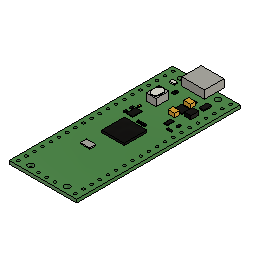
Raspberry+Pi+Pico (Autodesk Fusion 360 design; units mm, degrees)
Autodesk Fusion 360 part; units mm, degrees
sketch "Sketch1" plane through (0, 0, 0) normal (0, 0, 1) x (1, 0, 0)
  point P0 (-8.0088, 19.3196)
  point P1 (-8.0088, -20.4887)
  constraint vertical P0 P1
sketch "Sketch2" plane through (0, 0, 0) normal (0, 0, 1) x (1, 0, 0)
  line L0 (-10.4385, 24.6601) -> (10.5024, 24.6601)
  line L1 (10.5024, 24.6601) -> (10.5024, -25.9245)
  line L2 (10.5024, -25.9245) -> (-10.4385, -25.9245)
  line L3 (-10.4385, -25.9245) -> (-10.4385, 24.6601)
  dimension "d1" = 20.941
  constraint horizontal L0
  constraint vertical L1
  constraint horizontal L2
  constraint vertical L3
  measures "d1" distance of L0.start L0.end
extrude "Extrude1" add sketch "Sketch2" along normal blind 1
extrude "Extrude2" add 1 faces at (3.5221, -25.9245, 0.6667) along direction (0, -1, 0) blind 0.1
extrude "Extrude3" add 1 faces at (3.5221, -26.0245, 0.6667) along direction (0, -1, 0) blind 0.1
sketch "Sketch3" plane through (0, 0, 1) normal (0, 0, 1) x (-1, 0, 0)
  line L0 (-10.5024, 26.1245) -> (-10.5024, -24.6601)
  line L1 (-10.5024, -24.6601) -> (10.4385, -24.6601)
  line L2 (10.4385, -24.6601) -> (10.4385, 26.1245)
  line L3 (10.4385, 26.1245) -> (-10.5024, 26.1245)
  line L4 (3.5791, -2.7776) -> (-3.425, -2.7776)
  line L5 (-3.425, -2.7776) -> (-3.425, 4.2707)
  line L6 (-3.425, 4.2707) -> (3.5791, 4.2707)
  line L7 (3.5791, 4.2707) -> (3.5791, -2.7776)
  constraint horizontal L4
  constraint vertical L5
  constraint horizontal L6
  constraint vertical L7
extrude "Extrude4" add sketch "Sketch3" along normal blind 0.5 contours L4 L5 L6 L7
sketch "Sketch4" plane through (0, 0, 1) normal (0, 0, 1) x (-1, 0, 0)
  line L0 (3.5791, 4.2707) -> (3.5791, -2.7776)
  line L1 (3.5791, -2.7776) -> (-3.425, -2.7776)
  line L2 (-3.425, -2.7776) -> (-3.425, 4.2707)
  line L3 (-3.425, 4.2707) -> (3.5791, 4.2707)
  line L4 (-10.5024, 26.1245) -> (-10.5024, -24.6601)
  line L5 (-10.5024, -24.6601) -> (10.4385, -24.6601)
  line L6 (10.4385, -24.6601) -> (10.4385, 26.1245)
  line L7 (10.4385, 26.1245) -> (-10.5024, 26.1245)
  circle A0 centre (-8.7965, 24.8249) radius 0.4145
  circle A1 centre (-8.7965, 22.288) radius 0.4145
  circle A2 centre (-8.7965, 19.7512) radius 0.4145
  circle A3 centre (-8.7965, 17.2144) radius 0.4145
  circle A4 centre (-8.7965, 14.6775) radius 0.4145
  circle A5 centre (-8.7965, 12.1407) radius 0.4145
  circle A6 centre (-8.7965, 9.6038) radius 0.4145
  circle A7 centre (-8.7965, 7.067) radius 0.4145
  circle A8 centre (-8.7965, 4.5301) radius 0.4145
  circle A9 centre (-8.7965, 1.9933) radius 0.4145
  circle A10 centre (-8.7965, -0.5435) radius 0.4145
  circle A11 centre (-8.7965, -3.0804) radius 0.4145
  circle A12 centre (-8.7965, -5.6172) radius 0.4145
  circle A13 centre (-8.7965, -8.1541) radius 0.4145
  circle A14 centre (-8.7965, -10.6909) radius 0.4145
  circle A15 centre (-8.7965, -13.2277) radius 0.4145
  circle A16 centre (-8.7965, -15.7646) radius 0.4145
  circle A17 centre (-8.7965, -18.3014) radius 0.4145
  circle A18 centre (-8.7965, -20.8383) radius 0.4145
  circle A19 centre (-8.7965, -23.3751) radius 0.4145
  dimension "d10" = 0.829
  dimension "d13" = 0
  dimension "d14" = -48.2
  measures "d10" diameter of A0
extrude "Extrude5" cut sketch "Sketch4" against normal blind 14 contours A0 | A1 | A2 | A3 | A4 | A5 | A6 | A7 | A8 | A9 | A10 | A11 | A12 | A13 | A14 | A15 | A16 | A17 | A18 | A19
sketch "Sketch5" plane through (0, 0, 1) normal (0, 0, 1) x (-1, 0, 0)
  circle A0 centre (-8.7965, -18.3014) radius 0.4145
  circle A1 centre (-8.7965, -8.1541) radius 0.4145
  circle A2 centre (-8.7965, 1.9933) radius 0.4145
  circle A3 centre (-8.7965, 14.6775) radius 0.4145
  circle A4 centre (-8.7965, 24.8249) radius 0.4145
  circle A5 centre (-8.7965, 22.288) radius 0.4145
  circle A6 centre (-8.7965, 12.1407) radius 0.4145
  circle A7 centre (-8.7965, -0.5435) radius 0.4145
  circle A8 centre (-8.7965, -10.6909) radius 0.4145
  circle A9 centre (-8.7965, -20.8383) radius 0.4145
  circle A10 centre (-8.7965, -15.7646) radius 0.4145
  circle A11 centre (-8.7965, -5.6172) radius 0.4145
  circle A12 centre (-8.7965, 7.067) radius 0.4145
  circle A13 centre (-8.7965, 17.2144) radius 0.4145
  circle A14 centre (-8.7965, 4.5301) radius 0.4145
  circle A15 centre (-8.7965, 19.7512) radius 0.4145
  circle A16 centre (-8.7965, 9.6038) radius 0.4145
  circle A17 centre (-8.7965, -3.0804) radius 0.4145
  circle A18 centre (-8.7965, -13.2277) radius 0.4145
  circle A19 centre (-8.7965, -23.3751) radius 0.4145
  line L0 (3.5791, 4.2707) -> (3.5791, -2.7776)
  line L1 (3.5791, -2.7776) -> (-3.425, -2.7776)
  line L2 (-3.425, -2.7776) -> (-3.425, 4.2707)
  line L3 (-3.425, 4.2707) -> (3.5791, 4.2707)
  line L4 (-10.5024, 26.1245) -> (-10.5024, -24.6601)
  line L5 (-10.5024, -24.6601) -> (10.4385, -24.6601)
  line L6 (10.4385, -24.6601) -> (10.4385, 26.1245)
  line L7 (10.4385, 26.1245) -> (-10.5024, 26.1245)
  circle A20 centre (8.9761, 24.8199) radius 0.4252
  circle A21 centre (8.9761, 22.283) radius 0.4252
  circle A22 centre (8.9761, 19.7462) radius 0.4252
  circle A23 centre (8.9761, 17.2093) radius 0.4252
  circle A24 centre (8.9761, 14.6725) radius 0.4252
  circle A25 centre (8.9761, 12.1357) radius 0.4252
  circle A26 centre (8.9761, 9.5988) radius 0.4252
  circle A27 centre (8.9761, 7.062) radius 0.4252
  circle A28 centre (8.9761, 4.5251) radius 0.4252
  circle A29 centre (8.9761, 1.9883) radius 0.4252
  circle A30 centre (8.9761, -0.5486) radius 0.4252
  circle A31 centre (8.9761, -3.0854) radius 0.4252
  circle A32 centre (8.9761, -5.6222) radius 0.4252
  circle A33 centre (8.9761, -8.1591) radius 0.4252
  circle A34 centre (8.9761, -10.6959) radius 0.4252
  circle A35 centre (8.9761, -13.2328) radius 0.4252
  circle A36 centre (8.9761, -15.7696) radius 0.4252
  circle A37 centre (8.9761, -18.3065) radius 0.4252
  circle A38 centre (8.9761, -20.8433) radius 0.4252
  circle A39 centre (8.9761, -23.3801) radius 0.4252
  dimension "d17" = 0.8503
  dimension "d20" = 0
  dimension "d21" = -48.2
  measures "d17" diameter of A20
extrude "Extrude6" cut sketch "Sketch5" against normal blind 1 contours A20 | A21 | A22 | A23 | A24 | A25 | A26 | A27 | A28 | A29 | A30 | A31 | A32 | A33 | A34 | A35 | A36 | A37 | A38 | A39
sketch "Sketch6" plane through (0, 0, 1) normal (0, 0, 1) x (-1, 0, 0)
  circle A0 centre (8.9761, -18.3065) radius 0.4252
  circle A1 centre (8.9761, -8.1591) radius 0.4252
  circle A2 centre (8.9761, 1.9883) radius 0.4252
  circle A3 centre (8.9761, 12.1357) radius 0.4252
  circle A4 centre (8.9761, 22.283) radius 0.4252
  circle A5 centre (8.9761, 19.7462) radius 0.4252
  circle A6 centre (8.9761, 9.5988) radius 0.4252
  circle A7 centre (8.9761, -0.5486) radius 0.4252
  circle A8 centre (8.9761, -10.6959) radius 0.4252
  circle A9 centre (8.9761, -20.8433) radius 0.4252
  circle A10 centre (8.9761, -15.7696) radius 0.4252
  circle A11 centre (8.9761, -5.6222) radius 0.4252
  circle A12 centre (8.9761, 4.5251) radius 0.4252
  circle A13 centre (8.9761, 14.6725) radius 0.4252
  circle A14 centre (8.9761, 24.8199) radius 0.4252
  circle A15 centre (8.9761, 17.2093) radius 0.4252
  circle A16 centre (8.9761, 7.062) radius 0.4252
  circle A17 centre (8.9761, -3.0854) radius 0.4252
  circle A18 centre (8.9761, -13.2328) radius 0.4252
  circle A19 centre (8.9761, -23.3801) radius 0.4252
  circle A20 centre (-8.7965, -18.3014) radius 0.4145
  circle A21 centre (-8.7965, -8.1541) radius 0.4145
  circle A22 centre (-8.7965, 1.9933) radius 0.4145
  circle A23 centre (-8.7965, 14.6775) radius 0.4145
  circle A24 centre (-8.7965, 24.8249) radius 0.4145
  circle A25 centre (-8.7965, 22.288) radius 0.4145
  circle A26 centre (-8.7965, 12.1407) radius 0.4145
  circle A27 centre (-8.7965, -0.5435) radius 0.4145
  circle A28 centre (-8.7965, -10.6909) radius 0.4145
  circle A29 centre (-8.7965, -20.8383) radius 0.4145
  circle A30 centre (-8.7965, -15.7646) radius 0.4145
  circle A31 centre (-8.7965, -5.6172) radius 0.4145
  circle A32 centre (-8.7965, 7.067) radius 0.4145
  circle A33 centre (-8.7965, 17.2144) radius 0.4145
  circle A34 centre (-8.7965, 4.5301) radius 0.4145
  circle A35 centre (-8.7965, 19.7512) radius 0.4145
  circle A36 centre (-8.7965, 9.6038) radius 0.4145
  circle A37 centre (-8.7965, -3.0804) radius 0.4145
  circle A38 centre (-8.7965, -13.2277) radius 0.4145
  circle A39 centre (-8.7965, -23.3751) radius 0.4145
  line L0 (3.5791, 4.2707) -> (3.5791, -2.7776)
  line L1 (3.5791, -2.7776) -> (-3.425, -2.7776)
  line L2 (-3.425, -2.7776) -> (-3.425, 4.2707)
  line L3 (-3.425, 4.2707) -> (3.5791, 4.2707)
  line L4 (-10.5024, 26.1245) -> (-10.5024, -24.6601)
  line L5 (-10.5024, -24.6601) -> (10.4385, -24.6601)
  line L6 (10.4385, -24.6601) -> (10.4385, 26.1245)
  line L7 (10.4385, 26.1245) -> (-10.5024, 26.1245)
  circle A40 centre (-5.6173, 24.1526) radius 0.8768
  circle A41 centre (5.7716, 24.1573) radius 0.8814
extrude "Extrude7" cut sketch "Sketch6" against normal blind 1 contours A40 | A41
sketch "Sketch7" plane through (0, 0, 1) normal (0, 0, 1) x (-1, 0, 0)
  circle A0 centre (-5.6173, 24.1526) radius 0.8768
  circle A1 centre (5.7716, 24.1573) radius 0.8814
  circle A2 centre (8.9761, -18.3065) radius 0.4252
  circle A3 centre (8.9761, -8.1591) radius 0.4252
  circle A4 centre (8.9761, 1.9883) radius 0.4252
  circle A5 centre (8.9761, 12.1357) radius 0.4252
  circle A6 centre (8.9761, 22.283) radius 0.4252
  circle A7 centre (8.9761, 19.7462) radius 0.4252
  circle A8 centre (8.9761, 9.5988) radius 0.4252
  circle A9 centre (8.9761, -0.5486) radius 0.4252
  circle A10 centre (8.9761, -10.6959) radius 0.4252
  circle A11 centre (8.9761, -20.8433) radius 0.4252
  circle A12 centre (8.9761, -15.7696) radius 0.4252
  circle A13 centre (8.9761, -5.6222) radius 0.4252
  circle A14 centre (8.9761, 4.5251) radius 0.4252
  circle A15 centre (8.9761, 14.6725) radius 0.4252
  circle A16 centre (8.9761, 24.8199) radius 0.4252
  circle A17 centre (8.9761, 17.2093) radius 0.4252
  circle A18 centre (8.9761, 7.062) radius 0.4252
  circle A19 centre (8.9761, -3.0854) radius 0.4252
  circle A20 centre (8.9761, -13.2328) radius 0.4252
  circle A21 centre (8.9761, -23.3801) radius 0.4252
  circle A22 centre (-8.7965, -18.3014) radius 0.4145
  circle A23 centre (-8.7965, -8.1541) radius 0.4145
  circle A24 centre (-8.7965, 1.9933) radius 0.4145
  circle A25 centre (-8.7965, 14.6775) radius 0.4145
  circle A26 centre (-8.7965, 24.8249) radius 0.4145
  circle A27 centre (-8.7965, 22.288) radius 0.4145
  circle A28 centre (-8.7965, 12.1407) radius 0.4145
  circle A29 centre (-8.7965, -0.5435) radius 0.4145
  circle A30 centre (-8.7965, -10.6909) radius 0.4145
  circle A31 centre (-8.7965, -20.8383) radius 0.4145
  circle A32 centre (-8.7965, -15.7646) radius 0.4145
  circle A33 centre (-8.7965, -5.6172) radius 0.4145
  circle A34 centre (-8.7965, 7.067) radius 0.4145
  circle A35 centre (-8.7965, 17.2144) radius 0.4145
  circle A36 centre (-8.7965, 4.5301) radius 0.4145
  circle A37 centre (-8.7965, 19.7512) radius 0.4145
  circle A38 centre (-8.7965, 9.6038) radius 0.4145
  circle A39 centre (-8.7965, -3.0804) radius 0.4145
  circle A40 centre (-8.7965, -13.2277) radius 0.4145
  circle A41 centre (-8.7965, -23.3751) radius 0.4145
  line L0 (3.5791, 4.2707) -> (3.5791, -2.7776)
  line L1 (3.5791, -2.7776) -> (-3.425, -2.7776)
  line L2 (-3.425, -2.7776) -> (-3.425, 4.2707)
  line L3 (-3.425, 4.2707) -> (3.5791, 4.2707)
  line L4 (-10.5024, 26.1245) -> (-10.5024, -24.6601)
  line L5 (-10.5024, -24.6601) -> (10.4385, -24.6601)
  line L6 (10.4385, -24.6601) -> (10.4385, 26.1245)
  line L7 (10.4385, 26.1245) -> (-10.5024, 26.1245)
  circle A42 centre (-5.6142, -22.6811) radius 0.8718
  circle A43 centre (5.7752, -22.6811) radius 0.8763
extrude "Extrude8" cut sketch "Sketch7" against normal blind 1 contours A42 | A43
sketch "Sketch8" plane through (0, 0, 1) normal (0, 0, 1) x (-1, 0, 0)
  circle A0 centre (5.7752, -22.6811) radius 0.8763
  circle A1 centre (-5.6142, -22.6811) radius 0.8718
  circle A2 centre (-5.6173, 24.1526) radius 0.8768
  circle A3 centre (5.7716, 24.1573) radius 0.8814
  circle A4 centre (8.9761, -18.3065) radius 0.4252
  circle A5 centre (8.9761, -8.1591) radius 0.4252
  circle A6 centre (8.9761, 1.9883) radius 0.4252
  circle A7 centre (8.9761, 12.1357) radius 0.4252
  circle A8 centre (8.9761, 22.283) radius 0.4252
  circle A9 centre (8.9761, 19.7462) radius 0.4252
  circle A10 centre (8.9761, 9.5988) radius 0.4252
  circle A11 centre (8.9761, -0.5486) radius 0.4252
  circle A12 centre (8.9761, -10.6959) radius 0.4252
  circle A13 centre (8.9761, -20.8433) radius 0.4252
  circle A14 centre (8.9761, -15.7696) radius 0.4252
  circle A15 centre (8.9761, -5.6222) radius 0.4252
  circle A16 centre (8.9761, 4.5251) radius 0.4252
  circle A17 centre (8.9761, 14.6725) radius 0.4252
  circle A18 centre (8.9761, 24.8199) radius 0.4252
  circle A19 centre (8.9761, 17.2093) radius 0.4252
  circle A20 centre (8.9761, 7.062) radius 0.4252
  circle A21 centre (8.9761, -3.0854) radius 0.4252
  circle A22 centre (8.9761, -13.2328) radius 0.4252
  circle A23 centre (8.9761, -23.3801) radius 0.4252
  circle A24 centre (-8.7965, -18.3014) radius 0.4145
  circle A25 centre (-8.7965, -8.1541) radius 0.4145
  circle A26 centre (-8.7965, 1.9933) radius 0.4145
  circle A27 centre (-8.7965, 14.6775) radius 0.4145
  circle A28 centre (-8.7965, 24.8249) radius 0.4145
  circle A29 centre (-8.7965, 22.288) radius 0.4145
  circle A30 centre (-8.7965, 12.1407) radius 0.4145
  circle A31 centre (-8.7965, -0.5435) radius 0.4145
  circle A32 centre (-8.7965, -10.6909) radius 0.4145
  circle A33 centre (-8.7965, -20.8383) radius 0.4145
  circle A34 centre (-8.7965, -15.7646) radius 0.4145
  circle A35 centre (-8.7965, -5.6172) radius 0.4145
  circle A36 centre (-8.7965, 7.067) radius 0.4145
  circle A37 centre (-8.7965, 17.2144) radius 0.4145
  circle A38 centre (-8.7965, 4.5301) radius 0.4145
  circle A39 centre (-8.7965, 19.7512) radius 0.4145
  circle A40 centre (-8.7965, 9.6038) radius 0.4145
  circle A41 centre (-8.7965, -3.0804) radius 0.4145
  circle A42 centre (-8.7965, -13.2277) radius 0.4145
  circle A43 centre (-8.7965, -23.3751) radius 0.4145
  line L0 (3.5791, 4.2707) -> (3.5791, -2.7776)
  line L1 (3.5791, -2.7776) -> (-3.425, -2.7776)
  line L2 (-3.425, -2.7776) -> (-3.425, 4.2707)
  line L3 (-3.425, 4.2707) -> (3.5791, 4.2707)
  line L4 (-10.5024, 26.1245) -> (-10.5024, -24.6601)
  line L5 (-10.5024, -24.6601) -> (10.4385, -24.6601)
  line L6 (10.4385, -24.6601) -> (10.4385, 26.1245)
  line L7 (10.4385, 26.1245) -> (-10.5024, 26.1245)
  circle A44 centre (-2.4417, 24.8384) radius 0.4303
  circle A45 centre (0.0875, 24.8217) radius 0.4265
  circle A46 centre (2.6066, 24.8384) radius 0.43
extrude "Extrude9" cut sketch "Sketch8" against normal blind 1 contours A44 | A45 | A46
sketch "Sketch9" plane through (0, 0, 1) normal (0, 0, 1) x (-1, 0, 0)
  circle A0 centre (2.6066, 24.8384) radius 0.43
  circle A1 centre (0.0875, 24.8217) radius 0.4265
  circle A2 centre (-2.4417, 24.8384) radius 0.4303
  circle A3 centre (5.7752, -22.6811) radius 0.8763
  circle A4 centre (-5.6142, -22.6811) radius 0.8718
  circle A5 centre (-5.6173, 24.1526) radius 0.8768
  circle A6 centre (5.7716, 24.1573) radius 0.8814
  circle A7 centre (8.9761, -18.3065) radius 0.4252
  circle A8 centre (8.9761, -8.1591) radius 0.4252
  circle A9 centre (8.9761, 1.9883) radius 0.4252
  circle A10 centre (8.9761, 12.1357) radius 0.4252
  circle A11 centre (8.9761, 22.283) radius 0.4252
  circle A12 centre (8.9761, 19.7462) radius 0.4252
  circle A13 centre (8.9761, 9.5988) radius 0.4252
  circle A14 centre (8.9761, -0.5486) radius 0.4252
  circle A15 centre (8.9761, -10.6959) radius 0.4252
  circle A16 centre (8.9761, -20.8433) radius 0.4252
  circle A17 centre (8.9761, -15.7696) radius 0.4252
  circle A18 centre (8.9761, -5.6222) radius 0.4252
  circle A19 centre (8.9761, 4.5251) radius 0.4252
  circle A20 centre (8.9761, 14.6725) radius 0.4252
  circle A21 centre (8.9761, 24.8199) radius 0.4252
  circle A22 centre (8.9761, 17.2093) radius 0.4252
  circle A23 centre (8.9761, 7.062) radius 0.4252
  circle A24 centre (8.9761, -3.0854) radius 0.4252
  circle A25 centre (8.9761, -13.2328) radius 0.4252
  circle A26 centre (8.9761, -23.3801) radius 0.4252
  circle A27 centre (-8.7965, -18.3014) radius 0.4145
  circle A28 centre (-8.7965, -8.1541) radius 0.4145
  circle A29 centre (-8.7965, 1.9933) radius 0.4145
  circle A30 centre (-8.7965, 14.6775) radius 0.4145
  circle A31 centre (-8.7965, 24.8249) radius 0.4145
  circle A32 centre (-8.7965, 22.288) radius 0.4145
  circle A33 centre (-8.7965, 12.1407) radius 0.4145
  circle A34 centre (-8.7965, -0.5435) radius 0.4145
  circle A35 centre (-8.7965, -10.6909) radius 0.4145
  circle A36 centre (-8.7965, -20.8383) radius 0.4145
  circle A37 centre (-8.7965, -15.7646) radius 0.4145
  circle A38 centre (-8.7965, -5.6172) radius 0.4145
  circle A39 centre (-8.7965, 7.067) radius 0.4145
  circle A40 centre (-8.7965, 17.2144) radius 0.4145
  circle A41 centre (-8.7965, 4.5301) radius 0.4145
  circle A42 centre (-8.7965, 19.7512) radius 0.4145
  circle A43 centre (-8.7965, 9.6038) radius 0.4145
  circle A44 centre (-8.7965, -3.0804) radius 0.4145
  circle A45 centre (-8.7965, -13.2277) radius 0.4145
  circle A46 centre (-8.7965, -23.3751) radius 0.4145
  line L0 (3.5791, 4.2707) -> (3.5791, -2.7776)
  line L1 (3.5791, -2.7776) -> (-3.425, -2.7776)
  line L2 (-3.425, -2.7776) -> (-3.425, 4.2707)
  line L3 (-3.425, 4.2707) -> (3.5791, 4.2707)
  line L4 (-10.5024, 26.1245) -> (-10.5024, -24.6601)
  line L5 (-10.5024, -24.6601) -> (10.4385, -24.6601)
  line L6 (10.4385, -24.6601) -> (10.4385, 26.1245)
  line L7 (10.4385, 26.1245) -> (-10.5024, 26.1245)
  line L8 (6.534, -20.7124) -> (5.0323, -20.7124)
  line L9 (5.0323, -20.7124) -> (5.0323, -19.72)
  line L10 (5.0323, -19.72) -> (6.534, -19.72)
  line L11 (6.534, -19.72) -> (6.534, -20.7124)
  line L12 (-5.1342, -19.8019) -> (-6.5875, -19.8019)
  line L13 (-6.5875, -19.8019) -> (-6.5875, -17.2853)
  line L14 (-6.5875, -17.2853) -> (-5.1342, -17.2853)
  line L15 (-5.1342, -17.2853) -> (-5.1342, -19.8019)
  line L16 (-4.8684, -15.4776) -> (-6.8356, -15.4776)
  line L17 (-6.8356, -15.4776) -> (-6.8356, -12.9964)
  line L18 (-6.8356, -12.9964) -> (-4.8684, -12.9964)
  line L19 (-4.8684, -12.9964) -> (-4.8684, -15.4776)
  line L20 (-1.5188, -15.4244) -> (-4.0177, -15.4244)
  line L21 (-4.0177, -15.4244) -> (-4.0177, -12.9787)
  line L22 (-4.0177, -12.9787) -> (-1.5188, -12.9787)
  line L23 (-1.5188, -12.9787) -> (-1.5188, -15.4244)
  line L24 (3.3305, -18.5569) -> (2.3847, -18.5569)
  line L25 (2.3847, -18.5569) -> (2.3847, -18.0651)
  line L26 (2.3847, -18.0651) -> (3.3305, -18.0651)
  line L27 (3.3305, -18.0651) -> (3.3305, -18.5569)
  line L28 (3.3873, -17.7057) -> (2.3847, -17.7057)
  line L29 (2.3847, -17.7057) -> (2.3847, -17.195)
  line L30 (2.3847, -17.195) -> (3.3873, -17.195)
  line L31 (3.3873, -17.195) -> (3.3873, -17.7057)
  line L32 (-2.2118, -18.5758) -> (-3.2522, -18.5758)
  line L33 (-3.2522, -18.5758) -> (-3.2522, -18.0084)
  line L34 (-3.2522, -18.0084) -> (-2.2118, -18.0084)
  line L35 (-2.2118, -18.0084) -> (-2.2118, -18.5758)
  line L36 (-6.4679, -9.8556) -> (-7.0354, -9.8556)
  line L37 (-7.0354, -9.8556) -> (-7.0354, -8.7963)
  line L38 (-7.0354, -8.7963) -> (-6.4679, -8.7963)
  line L39 (-6.4679, -8.7963) -> (-6.4679, -9.8556)
  line L40 (-3.7251, -9.8556) -> (-4.7844, -9.8556)
  line L41 (-4.7844, -9.8556) -> (-4.7844, -7.7749)
  line L42 (-4.7844, -7.7749) -> (-3.7251, -7.7749)
  line L43 (-3.7251, -7.7749) -> (-3.7251, -9.8556)
  line L44 (4.8402, -7.5586) -> (2.8739, -7.5586)
  line L45 (2.8739, -7.5586) -> (2.8739, -4.6185)
  line L46 (2.8739, -4.6185) -> (4.8402, -4.6185)
  line L47 (4.8402, -4.6185) -> (4.8402, -7.5586)
  line L48 (3.8571, 8.6702) -> (0.9529, 8.6702)
  line L49 (0.9529, 8.6702) -> (0.9529, 10.5945)
  line L50 (0.9529, 10.5945) -> (3.8571, 10.5945)
  line L51 (3.8571, 10.5945) -> (3.8571, 8.6702)
  line L52 (-1.7197, -17.4888) -> (-3.782, -17.4888)
  line L53 (-3.782, -17.4888) -> (-3.782, -15.9462)
  line L54 (-3.782, -15.9462) -> (-1.7197, -15.9462)
  line L55 (-1.7197, -15.9462) -> (-1.7197, -17.4888)
  line L56 (-1.7197, -12.5929) -> (-3.782, -12.5929)
  line L57 (-3.782, -12.5929) -> (-3.782, -11.0336)
  line L58 (-3.782, -11.0336) -> (-1.7197, -11.0336)
  line L59 (-1.7197, -11.0336) -> (-1.7197, -12.5929)
  line L60 (-5.6582, -7.1654) -> (-7.1244, -7.1654)
  line L61 (-7.1244, -7.1654) -> (-7.1244, -6.6232)
  line L62 (-7.1244, -6.6232) -> (-5.6582, -6.6232)
  line L63 (-5.6582, -6.6232) -> (-5.6582, -7.1654)
  line L64 (5.8526, -7.6118) -> (5.3354, -7.6118)
  line L65 (5.3354, -7.6118) -> (5.3354, -6.5727)
  line L66 (5.3354, -6.5727) -> (5.8526, -6.5727)
  line L67 (5.8526, -6.5727) -> (5.8526, -7.6118)
  line L68 (4.911, -8.8608) -> (4.4817, -8.8608)
  line L69 (4.4817, -8.8608) -> (4.4817, -8.0802)
  line L70 (4.4817, -8.0802) -> (4.911, -8.0802)
  line L71 (4.911, -8.0802) -> (4.911, -8.8608)
  line L72 (5.8428, -5.6018) -> (5.3501, -5.6018)
  line L73 (5.3501, -5.6018) -> (5.3501, -4.626)
  line L74 (5.3501, -4.626) -> (5.8428, -4.626)
  line L75 (5.8428, -4.626) -> (5.8428, -5.6018)
  line L76 (1.0477, -4.7159) -> (0.6703, -4.7159)
  line L77 (0.6703, -4.7159) -> (0.6703, -3.9309)
  line L78 (0.6703, -3.9309) -> (1.0477, -3.9309)
  line L79 (1.0477, -3.9309) -> (1.0477, -4.7159)
  line L80 (0.3458, -4.7159) -> (-0.0392, -4.7159)
  line L81 (-0.0392, -4.7159) -> (-0.0392, -3.9309)
  line L82 (-0.0392, -3.9309) -> (0.3458, -3.9309)
  line L83 (0.3458, -3.9309) -> (0.3458, -4.7159)
  line L84 (-0.3411, -4.7159) -> (-0.7788, -4.7159)
  line L85 (-0.7788, -4.7159) -> (-0.7788, -3.9234)
  line L86 (-0.7788, -3.9234) -> (-0.3411, -3.9234)
  line L87 (-0.3411, -3.9234) -> (-0.3411, -4.7159)
  line L88 (-1.0656, -4.7159) -> (-1.4883, -4.7159)
  line L89 (-1.4883, -4.7159) -> (-1.4883, -3.9158)
  line L90 (-1.4883, -3.9158) -> (-1.0656, -3.9158)
  line L91 (-1.0656, -3.9158) -> (-1.0656, -4.7159)
  line L92 (5.1312, -15.1542) -> (2.1003, -15.1542)
  line L93 (2.1003, -15.1542) -> (2.1003, -11.1298)
  line L94 (2.1003, -11.1298) -> (5.1312, -11.1298)
  line L95 (5.1312, -11.1298) -> (5.1312, -15.1542)
  dimension "d30" = 1.5017
  dimension "d31" = 1.9672
  dimension "d32" = 2.4989
  dimension "d33" = 0.9458
  constraint horizontal L8
  constraint vertical L9
  constraint horizontal L10
  constraint vertical L11
  constraint horizontal L12
  constraint vertical L13
  constraint horizontal L14
  constraint vertical L15
  constraint horizontal L16
  constraint vertical L17
  constraint horizontal L18
  constraint vertical L19
  constraint horizontal L20
  constraint vertical L21
  constraint horizontal L22
  constraint vertical L23
  constraint horizontal L24
  constraint vertical L25
  constraint horizontal L26
  constraint vertical L27
  constraint horizontal L28
  constraint vertical L29
  constraint horizontal L30
  constraint vertical L31
  constraint horizontal L32
  constraint vertical L33
  constraint horizontal L34
  constraint vertical L35
  constraint horizontal L36
  constraint vertical L37
  constraint horizontal L38
  constraint vertical L39
  constraint horizontal L40
  constraint vertical L41
  constraint horizontal L42
  constraint vertical L43
  constraint horizontal L44
  constraint vertical L45
  constraint horizontal L46
  constraint vertical L47
  constraint horizontal L48
  constraint vertical L49
  constraint horizontal L50
  constraint vertical L51
  constraint horizontal L52
  constraint vertical L53
  constraint horizontal L54
  constraint vertical L55
  constraint horizontal L56
  constraint vertical L57
  constraint horizontal L58
  constraint vertical L59
  constraint horizontal L60
  constraint vertical L61
  constraint horizontal L62
  constraint vertical L63
  constraint horizontal L64
  constraint vertical L65
  constraint horizontal L66
  constraint vertical L67
  constraint horizontal L68
  constraint vertical L69
  constraint horizontal L70
  constraint vertical L71
  constraint horizontal L72
  constraint vertical L73
  constraint horizontal L74
  constraint vertical L75
  constraint horizontal L76
  constraint vertical L77
  constraint horizontal L78
  constraint vertical L79
  constraint horizontal L80
  constraint vertical L81
  constraint horizontal L82
  constraint vertical L83
  constraint horizontal L84
  constraint vertical L85
  constraint horizontal L86
  constraint vertical L87
  constraint horizontal L88
  constraint vertical L89
  constraint horizontal L90
  constraint vertical L91
  constraint horizontal L92
  constraint vertical L93
  constraint horizontal L94
  constraint vertical L95
  measures "d30" distance of L8.start L8.end
  measures "d31" distance of L16.start L16.end
  measures "d32" distance of L20.start L20.end
  measures "d33" distance of L24.start L24.end
extrude "Extrude10" add sketch "Sketch9" along normal blind 0.2 contours L24 L25 L26 L27 | L28 L29 L30 L31 | L32 L33 L34 L35 | L36 L37 L38 L39 | L40 L41 L42 L43 | L44 L45 L46 L47 | L60 L61 L62 L63 | L64 L65 L66 L67 | L72 L73 L74 L75 | L76 L77 L78 L79 | L80 L81 L82 L83 | L84 L85 L86 L87 | L88 L89 L90 L91
extrude "Extrude12" add sketch "Sketch9" along normal blind 0.5 contours L92 L93 L94 L95
extrude "Extrude13" add sketch "Sketch9" along normal blind 0.3 contours L12 L13 L14 L15 | L16 L17 L18 L19 | L20 L21 L22 L23 | L52 L53 L54 L55 | L56 L57 L58 L59
extrude "Extrude14" add sketch "Sketch9" along normal blind 0.35 contours L8 L9 L10 L11 | L48 L49 L50 L51 | L68 L69 L70 L71
sketch "Sketch10" plane through (0, 0, 1.5) normal (0, 0, 1) x (-1, 0, 0)
  line L0 (5.1312, -11.1298) -> (2.1003, -11.1298)
  line L1 (2.1003, -11.1298) -> (2.1003, -15.1542)
  line L2 (2.1003, -15.1542) -> (5.1312, -15.1542)
  line L3 (5.1312, -15.1542) -> (5.1312, -11.1298)
  line L4 (3.6329, -11.3187) -> (3.5869, -11.3187)
  line L5 (4.8869, -12.6187) -> (4.8869, -13.6585)
  line L6 (3.5869, -14.9585) -> (3.7329, -14.9585)
  line L7 (2.4329, -13.6585) -> (2.4329, -12.5187)
  arc A0 (3.6329, -11.3187) -> (2.4329, -12.5187) centre (3.6329, -12.5187) ccw
  arc A1 (4.8869, -12.6187) -> (3.5869, -11.3187) centre (3.5869, -12.6187) ccw
  arc A2 (2.4329, -13.6585) -> (3.7329, -14.9585) centre (3.7329, -13.6585) ccw
  arc A3 (3.5869, -14.9585) -> (4.8869, -13.6585) centre (3.5869, -13.6585) ccw
  dimension "d44" = 1.2
  dimension "d45" = 1.3
  dimension "d46" = 1.3
  dimension "d47" = 1.3
  constraint horizontal L4
  constraint vertical L5
  constraint horizontal L6
  constraint vertical L7
  constraint tangent L4 A0
  constraint tangent L7 A0
  constraint tangent L4 A1
  constraint tangent L5 A1
  constraint tangent L6 A2
  constraint tangent L7 A2
  constraint tangent L5 A3
  constraint tangent L6 A3
  measures "d44" radius of A0
  measures "d45" radius of A1
  measures "d46" radius of A2
  measures "d47" radius of A3
extrude "Extrude15" add sketch "Sketch10" along normal blind 0.5 contours L4 L5 L7 A0 A1 A2 A3
sketch "Sketch11" plane through (0, 0, 1) normal (0, 0, 1) x (-1, 0, 0)
  line L0 (3.6391, -26.7085) -> (-3.4408, -26.7085)
  line L1 (-3.4408, -26.7085) -> (-3.4408, -20.6681)
  line L2 (-3.4408, -20.6681) -> (3.6391, -20.6681)
  line L3 (3.6391, -20.6681) -> (3.6391, -26.7085)
  constraint horizontal L0
  constraint vertical L1
  constraint horizontal L2
  constraint vertical L3
extrude "Extrude16" add sketch "Sketch11" along normal blind 2
sketch "Sketch12" plane through (0, 26.7085, 0) normal (0, 1, 0) x (-1, 0, 0)
  line L0 (-3.4408, 1) -> (3.6391, 1)
  line L1 (3.6391, 1) -> (3.6391, 3)
  line L2 (3.6391, 3) -> (-3.4408, 3)
  line L3 (-3.4408, 3) -> (-3.4408, 1)
  line L4 (3.0663, 1.4632) -> (-3.0278, 1.4632)
  line L5 (-3.0278, 1.4632) -> (-3.0278, 2.5207)
  line L6 (-3.0278, 2.5207) -> (3.0663, 2.5207)
  line L7 (3.0663, 2.5207) -> (3.0663, 1.4632)
  constraint horizontal L4
  constraint vertical L5
  constraint horizontal L6
  constraint vertical L7
extrude "Extrude17" cut sketch "Sketch12" against normal blind 2 contours L4 L5 L6 L7
extrude "Extrude18" add 1 faces at (1.0808, 22.6816, 3) along direction (0, 0, 1) blind 0.5
extrude "Extrude19" cut 1 faces at (0.9965, 26.0418, 2.5207) along direction (0, 0, 1) blind 0.5
extrude "Extrude20" add 1 faces at (-1.2444, 0.4282, 1.5) along direction (0, 0, 1) blind 0.15
extrude "Extrude21" add 1 faces at (-2.2112, 12.9342, 1.5) along direction (0, 0, 1) blind 1.7
extrude "Extrude22" add 1 faces at (-3.2509, 12.932, 2) along direction (0, 0, 1) blind 2
extrude "Extrude23" cut 1 faces at (-3.2509, 12.932, 4) along direction (0, 0, -1) blind 0.6
extrude "Extrude24" add 1 faces at (2.4071, 16.9746, 1.3) along direction (0, 0, 1) blind 0.9
extrude "Extrude25" add 1 faces at (2.4071, 11.5533, 1.3) along direction (0, 0, 1) blind 0.9
extrude "Extrude26" add 1 faces at (6.1798, 13.8234, 1.3) along direction (0, 0, 1) blind 0.8
extrude "Extrude11" [suppressed]
